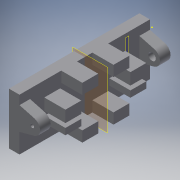
# Autodesk Inventor part: Assembly-jig-base
Saved by Autodesk Inventor 2018 (Build 220112000, 112)
## iProperties
Created: 2017-11-08
Part Number: Assembly-jig-base
Material: Generic
Document SubType Name: Modeling
Designer: xl0
Density: 1 g/cm^3
Appearance: Default
Author: xl0
Autodesk Inventor part; units mm, degrees
ref_plane "YZ Plane" through (0, 0, 0) normal (1, 0, 0) x (0, 1, 0)
ref_plane "XZ Plane" through (0, 0, 0) normal (0, 1, 0) x (-1, 0, 0)
ref_plane "XY Plane" through (0, 0, 0) normal (0, 0, 1) x (1, 0, 0)
ref_plane "Work Plane3" through (-2, 0, -40) normal (-1, 0, 0) x (0, 0, 1)
sketch "Sketch3" plane through (-2, 0, -8) normal (-1, 0, 0) x (0, -1, 0)
  line L0 (18.5447, 13.5) -> (31.5447, 13.5)
  line L1 (31.5447, 13.5) -> (31.5447, 3.5)
  line L2 (31.5447, 3.5) -> (18.5447, 3.5)
  line L3 (18.5447, 3.5) -> (18.5447, 13.5)
  line L4 (46.0447, 13.5) -> (59.0447, 13.5)
  line L5 (59.0447, 13.5) -> (59.0447, 3.5)
  line L6 (59.0447, 3.5) -> (46.0447, 3.5)
  line L7 (46.0447, 3.5) -> (46.0447, 13.5)
  line L8 (18.5447, -25.5) -> (31.5447, -25.5)
  line L9 (31.5447, -25.5) -> (31.5447, -35.5)
  line L10 (31.5447, -35.5) -> (18.5447, -35.5)
  line L11 (18.5447, -35.5) -> (18.5447, -25.5)
  line L12 (46.0447, -25.5) -> (59.0447, -25.5)
  line L13 (59.0447, -25.5) -> (59.0447, -35.5)
  line L14 (59.0447, -35.5) -> (46.0447, -35.5)
  line L15 (46.0447, -35.5) -> (46.0447, -25.5)
  line L16 (-2.9553, -32) -> (-2.9553, 8) projected
  line L17 (80.5447, 8) -> (80.5447, -32) projected
  line L18 (18.5447, 0) -> (18.5447, 3) projected
  line L19 (23.0447, 0) -> (23.0447, 3) projected
  line L20 (54.5447, 0) -> (54.5447, 3) projected
  line L21 (59.0447, 0) -> (59.0447, 3) projected
  line L22 (0.0447, 3) -> (77.5447, 3) projected
  line L23 (77.5447, -25) -> (0.0447, -25) projected
  line L24 (0.5447, -0.5) -> (13.5447, -0.5)
  line L25 (13.5447, -0.5) -> (13.5447, -11.5)
  line L26 (13.5447, -11.5) -> (0.5447, -11.5)
  line L27 (0.5447, -11.5) -> (0.5447, -0.5)
  line L28 (0.5447, -15.5) -> (13.5447, -15.5)
  line L29 (13.5447, -15.5) -> (13.5447, -21.5)
  line L30 (13.5447, -21.5) -> (0.5447, -21.5)
  line L31 (0.5447, -21.5) -> (0.5447, -15.5)
  line L32 (64.0447, -0.5) -> (77.0447, -0.5)
  line L33 (77.0447, -0.5) -> (77.0447, -11.5)
  line L34 (77.0447, -11.5) -> (64.0447, -11.5)
  line L35 (64.0447, -11.5) -> (64.0447, -0.5)
  line L36 (64.0447, -15.5) -> (77.0447, -15.5)
  line L37 (77.0447, -15.5) -> (77.0447, -21.5)
  line L38 (77.0447, -21.5) -> (64.0447, -21.5)
  line L39 (64.0447, -21.5) -> (64.0447, -15.5)
  line L40 (0.0447, 0) -> (77.5447, 0) projected
  line L41 (0.0447, -12) -> (77.5447, -12) projected
  line L42 (0.0447, -15) -> (77.5447, -15) projected
  line L43 (0.0447, -22) -> (77.5447, -22) projected
  line L44 (0.0447, -32) -> (0.0447, 8) projected
  line L45 (77.5447, 8) -> (77.5447, -32) projected
  point P0 (0, 8)
  dimension "d7" = 10
  dimension "d8" = 0.5
  dimension "d9" = 0.5
  dimension "d10" = 0.5
  dimension "d11" = 0.5
  dimension "d12" = 0.5
  dimension "d13" = 0.5
  dimension "d33" = 0.5
  dimension "d34" = 0.5
  dimension "d35" = 5
  dimension "d36" = 13
  dimension "d37" = 5
  constraints: 64 end point, 16 parallel, 13 collinear, 8 horizontal, 8 perpendicular, 4 equal length, 3 point on line, 1 other
  measures "d7" distance of L0.end L1.end
  measures "d8" distance between parallel lines of L2 L22
  measures "d9" distance between parallel lines of L23 L8
  measures "d10" distance between parallel lines of L26 L41
  measures "d11" distance between parallel lines of L40 L24
  measures "d12" distance between parallel lines of L42 L28
  measures "d13" distance between parallel lines of L43 L30
  measures "d34" distance between parallel lines of L37 L45
  measures "d35" distance between parallel lines of L3 L25
  measures "d36" distance of L9.end L10.end
  measures "d37" distance between parallel lines of L5 L35
extrude "Extrusion2" add sketch "Sketch3" against normal blind 20 contours L0 L1 L2 L3 | L4 L5 L6 L7 | L8 L9 L10 L11 | L12 L13 L14 L15 | L24 L25 L26 L27 | L28 L29 L30 L31 | L32 L33 L34 L35 | L36 L37 L38 L39
sketch "Sketch4" plane through (-2, 0, -8) normal (-1, 0, 0) x (0, 0, 1)
  line L0 (13.5, 22.9553) -> (-35.5, 22.9553)
  line L1 (-35.5, 22.9553) -> (-35.5, -100.5447)
  line L2 (-35.5, -100.5447) -> (13.5, -100.5447)
  line L3 (13.5, -100.5447) -> (13.5, 22.9553)
  line L4 (13.5, -18.5447) -> (13.5, -31.5447) projected
  line L5 (3.5, -18.5447) -> (13.5, -18.5447) projected
  line L6 (3.5, -31.5447) -> (3.5, -18.5447) projected
  line L7 (13.5, -31.5447) -> (3.5, -31.5447) projected
  line L8 (13.5, -46.0447) -> (13.5, -59.0447) projected
  line L9 (3.5, -46.0447) -> (13.5, -46.0447) projected
  line L10 (3.5, -59.0447) -> (3.5, -46.0447) projected
  line L11 (13.5, -59.0447) -> (3.5, -59.0447) projected
  line L12 (-25.5, -18.5447) -> (-25.5, -31.5447) projected
  line L13 (-35.5, -18.5447) -> (-25.5, -18.5447) projected
  line L14 (-35.5, -31.5447) -> (-35.5, -18.5447) projected
  line L15 (-25.5, -31.5447) -> (-35.5, -31.5447) projected
  line L16 (-25.5, -46.0447) -> (-25.5, -59.0447) projected
  line L17 (-35.5, -46.0447) -> (-25.5, -46.0447) projected
  line L18 (-35.5, -59.0447) -> (-35.5, -46.0447) projected
  line L19 (-25.5, -59.0447) -> (-35.5, -59.0447) projected
  line L20 (-32, 2.9553) -> (8, 2.9553) projected
  line L21 (8, -80.5447) -> (-32, -80.5447) projected
  line L22 (13.5, -18.5447) -> (13.5, -31.5447) projected
  line L23 (-35.5, -31.5447) -> (-35.5, -18.5447) projected
  point P0 (8, 0)
  dimension "d16" = 20
  dimension "d17" = 20
  constraints: 8 end point, 2 collinear, 2 parallel, 1 horizontal, 1 perpendicular
  measures "d16" distance between parallel lines of L0 L20
  measures "d17" distance between parallel lines of L2 L21
extrude "Extrusion3" add sketch "Sketch4" along normal blind 10
sketch "Sketch5" plane through (-2, 22.9553, 5.5) normal (0, 1, 0) x (1, 0, 0)
  point P0 (2, 5.5)
sketch "Sketch6" plane through (-2, 22.9553, 5.5) normal (0, 1, 0) x (1, 0, 0)
  line L0 (26.75, 28.5) -> (18.75, 28.5) projected
  line L1 (18.75, 28.5) -> (18.75, 25.5) projected
  line L2 (26.75, 25.5) -> (18.75, 25.5) projected
  line L3 (26.75, 28.5) -> (26.75, 25.5) projected
  line L4 (26.75, 13.5) -> (18.75, 13.5) projected
  line L5 (18.75, 13.5) -> (18.75, 10.5) projected
  line L6 (26.75, 10.5) -> (18.75, 10.5) projected
  line L7 (26.75, 13.5) -> (26.75, 10.5) projected
  arc A0 (13.9411, 12.2556) -> (13.9411, 26.7444) centre (12, 19.5) ccw
  line L8 (20, 25) -> (20, 14) projected
  line L9 (0, 0) -> (0, 49) projected
  line L10 (13.9411, 26.7444) -> (0, 30.48)
  line L11 (0, 29) -> (0, 35) projected
  line L12 (13.9411, 12.2556) -> (0, 8.52)
  line L13 (0, 49) -> (0, 0) projected
  point P0 (2, 5.5)
  point P1 (20, 19.5)
  dimension "d20" = 8
  dimension "d21" = 15
  dimension "d22" = 75
  dimension "d23" = 75
  constraints: 4 end point, 2 point on circle, 2 point on line, 2 tangent, 1 centre point, 1 horizontal alignment, 1 midpoint
  measures "d20" distance from line of A0.centre L8
  measures "d21" diameter of A0
  measures "d22" angle of L13 L10
  measures "d23" angle of L9 L12
extrude "Extrusion4" add sketch "Sketch6" against normal blind 10 contours L12 L9 L10 A0
sketch "Sketch7" plane through (-2, 12.9553, 5.5) normal (0, -1, 0) x (1, 0, 0)
  arc A0 (13.9411, -26.7444) -> (13.9411, -12.2556) centre (12, -19.5) ccw projected
  line L0 (0, -8.52) -> (13.9411, -12.2556) projected
  line L1 (13.9411, -26.7444) -> (0, -30.48) projected
  point P0 (2, -5.5)
hole "Hole1" at (10, 12.9553, -14) direction (0, 1, 0) diameter 3.5 end through all counterbore diameter 7 counterbore depth 5
ref_plane "Work Plane4" through (18, -38.7947, -4.5) normal (0, -1, 0) x (1, 0, 0)
sketch "Sketch8" plane through (18, -31.5447, 5.5) normal (0, 0, 1) x (1, 0, 0)
  line L0 (-20, 54.5) -> (-20, 13) projected
  line L1 (-20, 18) -> (-18.5, 18)
  line L2 (-18.5, 18) -> (-18.5, 13)
  line L3 (-18.5, 13) -> (-20, 13)
  line L4 (-20, 18) -> (0, 18) projected
  line L5 (-20, 13) -> (0, 13) projected
  line L6 (-20, 18) -> (-9.8118, 18) construction
  line L7 (-20, 13) -> (-11.1239, 13) construction
  line L8 (-20, 13) -> (0, 13) construction
  line L9 (-20.8217, 15.5) -> (-11.5802, 15.5) construction
  point P0 (-18, 31.5447)
  dimension "d38" = 1.5
  dimension "d39" = 5
  constraints: 12 end point, 4 point on line, 3 perpendicular, 1 horizontal, 2 other
  measures "d38" distance between parallel lines of L0 L2
  measures "d39" distance between parallel lines of L3 L1
extrude "Extrusion5" add sketch "Sketch8" against normal up to surface (49 mm away)
mirror "Mirror1" about plane through (18, -38.7947, -4.5) normal (0, -1, 0) of "Extrusion4", "Hole1", "Extrusion5"
sketch "Sketch9" plane through (-2, -90.5447, -3.02) normal (0, 1, 0) x (1, 0, 0)
  line L0 (0, 5.48) -> (0, -8.52) projected
  line L1 (0, 40.48) -> (0, 26.48) projected
  line L2 (0, 1.48) -> (0, -8.52) projected
  line L3 (0, 30.48) -> (0, 40.48) projected
  line L4 (1.5, -8.52) -> (1.5, 5.48) projected
  line L5 (1.5, 26.48) -> (1.5, 40.48) projected
  line L6 (0, -6.02) -> (1.5, -6.02)
  line L7 (1.5, -8.52) -> (1.5, 1.48) projected
  line L8 (1.5, -1.02) -> (0, -1.02)
  line L9 (1.5, 30.48) -> (1.5, 40.48) projected
  line L10 (1.5, 32.98) -> (0, 32.98)
  line L11 (1.5, 37.98) -> (0, 37.98)
  line L12 (2, 1.98) -> (18.75, 1.98) projected
  line L13 (9.75, 29.98) -> (2, 29.98) projected
  line L14 (1.5, 1.48) -> (20, 1.48) projected
  line L15 (1.5, 30.48) -> (20, 30.48) projected
  point P0 (2, -3.02)
  dimension "d42" = 2.5
  dimension "d43" = 2.5
  dimension "d44" = 5
  dimension "d45" = 5
  constraints: 8 end point, 8 point on line, 4 perpendicular
  measures "d42" distance between parallel lines of L14 L8
  measures "d43" distance between parallel lines of L10 L15
  measures "d44" distance between parallel lines of L8 L6
  measures "d45" distance between parallel lines of L11 L10
extrude "Extrusion6" add sketch "Sketch9" along normal blind 20
mirror "Mirror2" about plane through (18, -38.7947, -4.5) normal (0, -1, 0) of "Extrusion6"
equation "\"d10\" = d8"
equation "\"d11\" = d8"
equation "\"d12\" = d8"
equation "\"d13\" = d8"
equation "\"d33\" = d9"
equation "\"d34\" = d9"
equation "\"d37\" = d35"
equation "\"d17\" = d16"
equation "\"d43\" = d42"
equation "\"d45\" = d44"
body "Solid2"
